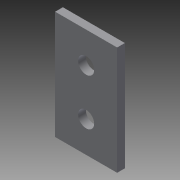
# Autodesk Inventor part: Chassis Tower Support Plate (for Bracket 1)
Saved by Autodesk Inventor 2013 (Build 170138000, 138)
## iProperties
Created: 2013-01-30
Part Number: Chassis Tower Support Plate (for Bracket 1)
Material: Generic
Document SubType Name: Modeling
Designer: Moses
Density: 1 g/cm^3
Author: Moses
Autodesk Inventor part; units mm, degrees
ref_plane "YZ Plane" through (0, 0, 0) normal (1, 0, 0) x (0, 1, 0)
ref_plane "XZ Plane" through (0, 0, 0) normal (0, 1, 0) x (-1, 0, 0)
ref_plane "XY Plane" through (0, 0, 0) normal (0, 0, 1) x (1, 0, 0)
sketch "Sketch1" plane through (0, 0, 0) normal (0, 0, 1) x (1, 0, 0)
  line L0 (0, 0) -> (25.4, 0)
  line L1 (25.4, 0) -> (25.4, 44.45)
  line L2 (25.4, 44.45) -> (0, 44.45)
  line L3 (0, 44.45) -> (0, 0)
  line L4 (12.7, 44.45) -> (12.7, 0) construction
  circle A0 centre (12.7, 31.75) radius 3.302
  circle A1 centre (12.7, 12.7) radius 3.302
  dimension "d0" = 25.4
  dimension "d2" = 44.45
  dimension "d3" = 6.604
  dimension "d4" = 19.05
  dimension "d5" = 12.7
  constraints: 10 end point, 2 centre point, 2 midpoint, 2 parallel, 2 point on line, 1 equal radius, 1 horizontal, 1 perpendicular
  measures "d0" distance of L1.end L2.end
  measures "d2" distance of L2.end L0.start
  measures "d3" diameter of A0
  measures "d4" distance of A1.centre A0.centre
  measures "d5" distance from line of L2 A0.centre
extrude "Extrusion1" add sketch "Sketch1" along normal blind 3.175
body "Solid1"
